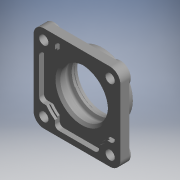
# Autodesk Inventor part: FY 506 M-housing
Saved by Autodesk Inventor 2017.3 (Build 213256000, 256)
## iProperties
Part Number: FY 506 M-housing
Material: Generic
Catalog Web Link: www.cadenas.de
Description: ayf_001hc_hh_hy-housing-Square flanged housings for Y-bearings
Vendor: SKF
Document SubType Name: Modeling
Designer: partserver
Manufacturer: SKF
Mass: 106.222 g
Surface Area: 357.74 cm^2
Volume: 106.222 cm^3
Density: 1 g/cm^3
Appearance: PSOLRGB-175-175-175
Category: PARTsolutions
Company: SKF
Title: FY 506 M-housing
Author: Cadenas PARTsolutions
Comments: Square flanged housings for Y-bearings
PSOL_IDENT_0: {$CADENAS_DATA\23d-libs\skf\bearings_units_and_housings\bearing_units\ball_bearing_units\y-units\y-b
PSOL_IDENT_1: earing_square_flanged_units_parts\ayf_001hc_hh_hy_housing.prj},196 {VTYP=3D},{NB=FY 506 M-housing},{
PSOL_IDENT_2: LINA=FY 506 M-housing},{NN=ayf_001hc_hh_hy-housing},{DATE=20.08.2020 13:45:19},{GEOMDATE=29.07.2020
PSOL_IDENT_3: 16:36:58},{VERSION=},{LINEID=8870},{WBVAR=COVER},{WBNUMERIC=}  {NB=FY 506 M-housing},{LINA=FY 506 M-
PSOL_IDENT_4: housing},{KT=DUMMY},{DESIGNATION=FY 506 M},{SS1=26.700},{T=46.700},{COVER=},{GN=1/4-28 SAE-LT},{D=62
PSOL_IDENT_5: .000},{DA=93.700},{DB1=76.000},{DB2=84.000},{DB=0.000},{A=32.500},{A1=13.000},{A2=20.000},{A3=3.200}
PSOL_IDENT_6: ,{A5=20.000},{J=82.500},{L=108.000},{N=11.500},{RG=1/4-28 UNF},{R1=21.000},{DN=6.500},{SWN=7.000},{J
PSOL_IDENT_7: 6=96.000},{J7=24.500},{N4=4.000},{EC=ECY 206},{AEC=25.000},{DEC=59.400},{D1EC=65.000},{D2EC=66.500},
PSOL_IDENT_8: {E=18},{DESIGN=fy},{BRG=0.000},{ECPN=},{H4=MIN},{R2=MIN},{R3=MIN},{R4=MIN},{L1=MIN},{H5=MIN},{R5=MIN
PSOL_IDENT_9: },{H6=MIN},{L2=MIN},{H7=MIN},{H8=MIN},{H9=MIN},{L3=MIN},{L4=MIN},{H10=MIN},{H11=MIN},{H12=MIN},{H13=
PSOL_IDENT_10: MIN},{H14=MIN},{R6=MIN},{L5=MIN},{H15=MIN},{H16=MIN},{SC=MIN}
NB: FY 506 M-housing
NN: ayf_001hc_hh_hy-housing
NT: Square flanged housings for Y-bearings
NBSYN: $DESIGNATION.$ECPN.-housing
LINA: FY 506 M-housing
CATALOG: SKF
DESIGNATION: FY 506 M
SS1: 26.7
T: 46.7
COVER: No End Cover
GN: 1/4-28 SAE-LT
D: 62
DA: 93.7
DB1: 76
DB2: 84
DB: 0
A: 32.5
A1: 13
A2: 20
A3: 3.2
A5: 20
J: 82.5
L: 108
N: 11.5
RG: 1/4-28 UNF
R1: 21
DN: 6.5
SWN: 7
J6: 96
J7: 24.5
N4: 4
EC: ECY 206
AEC: 25
DEC: 59.4
D1EC: 65
D2EC: 66.5
DESIGN: fy
H4: 0
R2: 0
R3: 0
R4: 0
L1: 0
H5: 0
R5: 0
H6: 0
L2: 0
H7: 0
H8: 0
H9: 0
L3: 0
L4: 0
H10: 0
H11: 0
H12: 0
H13: 0
H14: 0
R6: 0
L5: 0
H15: 0
H16: 0
SC: 0
SUPPLIER: SKF
ARTICLENO: FY 506 M-housing
BOMINFO: FY 506 M-housing
CREATOR: CADENAS GmbH
Autodesk Inventor part; units mm, degrees
sketch "Sketch_1" plane through (0, 0, 0) normal (0, 0, 1) x (1, 0, 0)
  line L0 (0, 0) -> (0, 32.5)
  line L1 (29.6648, 9) -> (32.6648, 6)
  line L2 (32.6648, 6) -> (44.991, 6)
  line L3 (44.991, 6) -> (44.991, 3.2)
  line L4 (44.991, 3.2) -> (46.85, 3.2)
  line L5 (46.85, 3.2) -> (46.85, 0)
  line L6 (46.85, 0) -> (76.3675, 0)
  line L7 (76.3675, 0) -> (76.3675, 11)
  line L8 (76.3675, 11) -> (45, 11)
  arc A0 (42.0754, 13.3318) -> (45, 11) centre (45, 14) ccw
  line L9 (42.0754, 13.3318) -> (37.9623, 31.3341)
  arc A1 (37.9623, 31.3341) -> (36.5, 32.5) centre (36.5, 31) ccw
  line L10 (36.5, 32.5) -> (31, 32.5)
  line L11 (31, 32.5) -> (31, 30.3352)
  line L12 (31, 30.3352) -> (29.6648, 29)
  arc A2 (29.6648, 11) -> (29.6648, 29) centre (0, 20) ccw
  line L13 (29.6648, 11) -> (29.6648, 9)
  constraints: 28 end point, 6 point on circle, 3 centre point
revolve "Revolution1" add sketch "Sketch_1" angle 360 about axis through (0, 0, 0) along (0, -1, 0)
sketch "Sketch_2" plane through (0, 11, 0) normal (0, 1, 0) x (1, 0, 0)
  arc A0 (-50.2656, -32.2344) -> (-32.2344, -50.2656) centre (-41.25, -41.25) ccw
  line L0 (-32.2344, -50.2656) -> (-19.2814, -37.3126)
  arc A1 (-19.2814, -37.3126) -> (19.2814, -37.3126) centre (0, 0) ccw
  line L1 (19.2814, -37.3126) -> (32.2344, -50.2656)
  arc A2 (32.2344, -50.2656) -> (50.2656, -32.2344) centre (41.25, -41.25) ccw
  line L2 (50.2656, -32.2344) -> (37.3126, -19.2814)
  arc A3 (37.3126, -19.2814) -> (37.3126, 19.2814) centre (0, 0) ccw
  line L3 (37.3126, 19.2814) -> (50.2656, 32.2344)
  arc A4 (50.2656, 32.2344) -> (32.2344, 50.2656) centre (41.25, 41.25) ccw
  line L4 (32.2344, 50.2656) -> (19.2814, 37.3126)
  arc A5 (19.2814, 37.3126) -> (-19.2814, 37.3126) centre (0, 0) ccw
  line L5 (-19.2814, 37.3126) -> (-32.2344, 50.2656)
  arc A6 (-32.2344, 50.2656) -> (-50.2656, 32.2344) centre (-41.25, 41.25) ccw
  line L6 (-50.2656, 32.2344) -> (-37.3126, 19.2814)
  arc A7 (-37.3126, 19.2814) -> (-37.3126, -19.2814) centre (0, 0) ccw
  line L7 (-37.3126, -19.2814) -> (-50.2656, -32.2344)
  circle A8 centre (0, 0) radius 41.5
  constraints: 16 end point, 16 point on circle, 9 centre point
extrude "Extrusion1" add sketch "Sketch_2" along normal blind 2
sketch "Sketch_3" plane through (0, 0, 0) normal (0, 1, 0) x (-1, 0, 0)
  line L0 (108, -108) -> (108, 108)
  line L1 (108, 108) -> (-108, 108)
  line L2 (-108, 108) -> (-108, -108)
  line L3 (-108, -108) -> (108, -108)
  arc A0 (54, 41.25) -> (41.25, 54) centre (41.25, 41.25) ccw
  line L4 (41.25, 54) -> (-41.25, 54)
  arc A1 (-41.25, 54) -> (-54, 41.25) centre (-41.25, 41.25) ccw
  line L5 (-54, 41.25) -> (-54, -41.25)
  arc A2 (-54, -41.25) -> (-41.25, -54) centre (-41.25, -41.25) ccw
  line L6 (-41.25, -54) -> (41.25, -54)
  arc A3 (41.25, -54) -> (54, -41.25) centre (41.25, -41.25) ccw
  line L7 (54, -41.25) -> (54, 41.25)
  constraints: 16 end point, 8 point on circle, 4 centre point
extrude "Extrusion2" cut sketch "Sketch_3" along normal blind 32.5
sketch "Sketch4" plane through (-41.25, 0, -54) normal (0, -1, 0) x (1, 0, 0)
  point P0 (0, 95.25)
hole "Hole1" at (-41.25, 0, 41.25) direction (0, 1, 0) diameter 11.5 depth 13
pattern_linear "Rectangular Pattern1" count 2 spacing 82.5 along (1, 0, 0) count 2 spacing 82.5 along (0, 0, -1) of "Hole1"
sketch "Sketch_8" plane through (0, 0, 0) normal (1, 0, 0) x (0, 1, 0)
  line L0 (21, -40.3234) -> (14.0953, -10.1021)
  line L1 (14.0953, -10.1021) -> (17.1905, -9.3949)
  line L2 (17.1905, -9.3949) -> (24.0952, -39.6162)
  line L3 (24.0952, -39.6162) -> (21, -40.3234)
  line L4 (21, -40.3234) -> (14.0953, -10.1021)
  constraints: 10 end point
revolve "Revolution2" cut sketch "Sketch_8" angle 360 about axis through (0, 21, -40.3234) along (0, 0.2227338, -0.9748793)
sketch "Sketch_6" plane through (0, 11, 0) normal (0, 1, 0) x (1, 0, 0)
  line L0 (-50, -24.5) -> (50, -24.5)
  arc A0 (-50, -24.5) -> (-46, -24.5) centre (-48, -24.5) ccw
  line L1 (-50, -24.5) -> (-46, -24.5)
  constraints: 4 end point, 2 point on circle, 1 centre point
revolve "Revolution3" cut sketch "Sketch_6" angle 360 about axis through (-50, 11, 24.5) along (-1, 0, 0)
sketch "Sketch_17" plane through (0, 0, 0) normal (0, 0, 1) x (1, 0, 0)
  line L0 (0, 0) -> (0, 32.5)
  line L1 (27, 26.8511) -> (27, 14.1493)
  line L2 (27, 14.1493) -> (33.5, 17.9021)
  arc A0 (33.5, 17.9021) -> (33.5, 23.0983) centre (32, 20.5002) ccw
  line L3 (33.5, 23.0983) -> (27, 26.8511)
  constraints: 8 end point, 2 point on circle, 1 centre point
revolve "Revolution4" cut sketch "Sketch_17" angle 360 about axis through (0, 0, 0) along (0, -1, 0)
sketch "Sketch_7" plane through (0, 20, 0) normal (0, 1, 0) x (1, 0, 0)
  arc A0 (-27.4003, 14.499) -> (-27.4003, -14.499) centre (0, 0) ccw
  line L0 (-27.4003, -14.499) -> (27.4003, -14.499)
  arc A1 (27.4003, -14.499) -> (27.4003, 14.499) centre (0, 0) ccw
  line L1 (27.4003, 14.499) -> (-27.4003, 14.499)
  constraints: 4 end point, 4 point on circle, 2 centre point
extrude "Extrusion3" cut sketch "Sketch_7" along normal blind 13.975
sketch "Sketch_11" plane through (0, 0, 0) normal (0, 1, 0) x (-1, 0, 0)
  arc A0 (47, 22.45) -> (42, 27.45) centre (42, 22.45) ccw
  line L0 (42, 27.45) -> (27.45, 27.45)
  line L1 (27.45, 27.45) -> (27.45, 42)
  arc A1 (27.45, 42) -> (22.45, 47) centre (22.45, 42) ccw
  line L2 (22.45, 47) -> (-22.45, 47)
  arc A2 (-22.45, 47) -> (-27.45, 42) centre (-22.45, 42) ccw
  line L3 (-27.45, 42) -> (-27.45, 27.45)
  line L4 (-27.45, 27.45) -> (-42, 27.45)
  arc A3 (-42, 27.45) -> (-47, 22.45) centre (-42, 22.45) ccw
  line L5 (-47, 22.45) -> (-47, -22.45)
  arc A4 (-47, -22.45) -> (-42, -27.45) centre (-42, -22.45) ccw
  line L6 (-42, -27.45) -> (-27.45, -27.45)
  line L7 (-27.45, -27.45) -> (-27.45, -42)
  arc A5 (-27.45, -42) -> (-22.45, -47) centre (-22.45, -42) ccw
  line L8 (-22.45, -47) -> (22.45, -47)
  arc A6 (22.45, -47) -> (27.45, -42) centre (22.45, -42) ccw
  line L9 (27.45, -42) -> (27.45, -27.45)
  line L10 (27.45, -27.45) -> (42, -27.45)
  arc A7 (42, -27.45) -> (47, -22.45) centre (42, -22.45) ccw
  line L11 (47, -22.45) -> (47, 22.45)
  constraints: 24 end point, 16 point on circle, 8 centre point
extrude "Extrusion4" cut sketch "Sketch_11" along normal blind 6
sketch "Sketch_12" plane through (0, 11, 0) normal (0, 1, 0) x (1, 0, 0)
  arc A0 (-52.5, 4.7066) -> (-52.2623, 4.4689) centre (-52.2623, 4.7066) ccw
  line L0 (-52.2623, 4.4689) -> (-50.6968, 4.4689)
  arc A1 (-50.6968, 4.4689) -> (-50.5287, 4.5385) centre (-50.6968, 4.7066) ccw
  line L1 (-50.5287, 4.5385) -> (-50.4595, 4.6077)
  arc A2 (-50.2207, 4.7066) -> (-50.4595, 4.6077) centre (-50.2207, 4.3689) ccw
  line L2 (-50.2207, 4.7066) -> (-49.0328, 4.7066)
  arc A3 (-48.8648, 4.637) -> (-49.0328, 4.7066) centre (-49.0328, 4.4689) ccw
  line L3 (-48.8648, 4.637) -> (-48.7663, 4.5385)
  arc A4 (-48.7663, 4.5385) -> (-48.5982, 4.4689) centre (-48.5982, 4.7066) ccw
  line L4 (-48.5982, 4.4689) -> (-47.2704, 4.4689)
  line L5 (-47.2704, 4.4689) -> (-47.2704, 3.732)
  line L6 (-47.2704, 3.732) -> (-48.6967, 3.732)
  arc A5 (-48.6967, 3.732) -> (-48.9344, 3.4943) centre (-48.6967, 3.4943) ccw
  line L7 (-48.9344, 3.4943) -> (-48.9344, 1.9183)
  arc A6 (-48.9916, 1.7636) -> (-48.9344, 1.9183) centre (-49.1721, 1.9183) ccw
  line L8 (-48.9916, 1.7636) -> (-50.3606, 0.1664)
  line L9 (-50.3606, 0.1664) -> (-51.0041, 0.8099)
  arc A7 (-51.0738, 0.978) -> (-51.0041, 0.8099) centre (-50.836, 0.978) ccw
  line L10 (-51.0738, 0.978) -> (-51.0738, 2.7812)
  arc A8 (-51.0738, 2.7812) -> (-51.3115, 3.0189) centre (-51.3115, 2.7812) ccw
  line L11 (-51.3115, 3.0189) -> (-52.2623, 3.0189)
  arc A9 (-52.2623, 3.0189) -> (-52.5, 2.7812) centre (-52.2623, 2.7812) ccw
  line L12 (-52.5, 2.7812) -> (-52.5, 0.7486)
  arc A10 (-52.5, 0.7486) -> (-52.4202, 0.5709) centre (-52.2623, 0.7486) ccw
  line L13 (-52.4202, 0.5709) -> (-50.3606, -1.2599)
  line L14 (-50.3606, -1.2599) -> (-52.2623, -1.2599)
  arc A11 (-52.2623, -1.2599) -> (-52.5, -1.4976) centre (-52.2623, -1.4976) ccw
  line L15 (-52.5, -1.4976) -> (-52.5, -3.3992)
  arc A12 (-52.5, -3.3992) -> (-52.2623, -3.6369) centre (-52.2623, -3.3992) ccw
  line L16 (-52.2623, -3.6369) -> (-50.6968, -3.6369)
  arc A13 (-50.6968, -3.6369) -> (-50.5287, -3.5673) centre (-50.6968, -3.3992) ccw
  line L17 (-50.5287, -3.5673) -> (-50.4302, -3.4689)
  arc A14 (-50.2622, -3.3992) -> (-50.4302, -3.4689) centre (-50.2622, -3.6369) ccw
  line L18 (-50.2622, -3.3992) -> (-49.2705, -3.3992)
  arc A15 (-49.1025, -3.4689) -> (-49.2705, -3.3992) centre (-49.2705, -3.6369) ccw
  line L19 (-49.1025, -3.4689) -> (-49.004, -3.5673)
  arc A16 (-49.004, -3.5673) -> (-48.8359, -3.6369) centre (-48.8359, -3.3992) ccw
  line L20 (-48.8359, -3.6369) -> (-47.2704, -3.6369)
  line L21 (-47.2704, -3.6369) -> (-47.2704, -4.1124)
  line L22 (-47.2704, -4.1124) -> (-50.1229, -4.1124)
  arc A17 (-50.1229, -4.1124) -> (-50.3606, -4.3501) centre (-50.1229, -4.3501) ccw
  line L23 (-50.3606, -4.3501) -> (-50.3606, -8.1534)
  arc A18 (-50.5983, -8.3911) -> (-50.3606, -8.1534) centre (-50.5983, -8.1534) ccw
  line L24 (-50.5983, -8.3911) -> (-51.5492, -8.3911)
  arc A19 (-51.7869, -8.1534) -> (-51.5492, -8.3911) centre (-51.5492, -8.1534) ccw
  line L25 (-51.7869, -8.1534) -> (-51.7869, -7.2026)
  arc A20 (-51.5492, -6.9649) -> (-51.7869, -7.2026) centre (-51.5492, -7.2026) ccw
  line L26 (-51.5492, -6.9649) -> (-51.3115, -6.9649)
  arc A21 (-51.3115, -6.9649) -> (-51.0738, -6.7271) centre (-51.3115, -6.7271) ccw
  line L27 (-51.0738, -6.7271) -> (-51.0738, -5.0632)
  arc A22 (-51.0738, -5.0632) -> (-51.3115, -4.8255) centre (-51.3115, -5.0632) ccw
  line L28 (-51.3115, -4.8255) -> (-52.1923, -4.8255)
  arc A23 (-52.1923, -4.8255) -> (-52.5, -5.1332) centre (-52.1923, -5.1332) ccw
  line L29 (-52.5, -5.1332) -> (-52.5, -10.2428)
  arc A24 (-52.5, -10.2428) -> (-52.2123, -10.5305) centre (-52.2123, -10.2428) ccw
  line L30 (-52.2123, -10.5305) -> (-49.8852, -10.5305)
  arc A25 (-49.8852, -10.5305) -> (-49.6475, -10.2928) centre (-49.8852, -10.2928) ccw
  line L31 (-49.6475, -10.2928) -> (-49.6475, -6.4894)
  arc A26 (-49.4098, -6.2517) -> (-49.6475, -6.4894) centre (-49.4098, -6.4894) ccw
  line L32 (-49.4098, -6.2517) -> (-47.7458, -6.2517)
  arc A27 (-47.5081, -6.4894) -> (-47.7458, -6.2517) centre (-47.7458, -6.4894) ccw
  line L33 (-47.5081, -6.4894) -> (-47.5081, -8.8665)
  arc A28 (-47.7458, -9.1042) -> (-47.5081, -8.8665) centre (-47.7458, -8.8665) ccw
  line L34 (-47.7458, -9.1042) -> (-48.6967, -9.1042)
  arc A29 (-48.6967, -9.1042) -> (-48.9344, -9.3419) centre (-48.6967, -9.3419) ccw
  line L35 (-48.9344, -9.3419) -> (-48.9344, -11.0059)
  arc A30 (-48.9344, -11.0059) -> (-48.6967, -11.2436) centre (-48.6967, -11.0059) ccw
  line L36 (-48.6967, -11.2436) -> (-47.0327, -11.2436)
  arc A31 (-47.0327, -11.2436) -> (-46.795, -11.0059) centre (-47.0327, -11.0059) ccw
  line L37 (-46.795, -11.0059) -> (-46.795, -4.3501)
  arc A32 (-46.795, -4.3501) -> (-47.0327, -4.1124) centre (-47.0327, -4.3501) ccw
  line L38 (-47.0327, -4.1124) -> (-47.0327, -3.6369)
  arc A33 (-47.0327, -3.6369) -> (-46.795, -3.3992) centre (-47.0327, -3.3992) ccw
  line L39 (-46.795, -3.3992) -> (-46.795, -1.4976)
  arc A34 (-46.795, -1.4976) -> (-47.0327, -1.2599) centre (-47.0327, -1.4976) ccw
  line L40 (-47.0327, -1.2599) -> (-48.9344, -1.2599)
  line L41 (-48.9344, -1.2599) -> (-46.8646, 0.8099)
  arc A35 (-46.8646, 0.8099) -> (-46.795, 0.978) centre (-47.0327, 0.978) ccw
  line L42 (-46.795, 0.978) -> (-46.795, 3.4943)
  arc A36 (-46.795, 3.4943) -> (-47.0327, 3.732) centre (-47.0327, 3.4943) ccw
  line L43 (-47.0327, 3.732) -> (-47.0327, 4.4689)
  arc A37 (-47.0327, 4.4689) -> (-46.795, 4.7066) centre (-47.0327, 4.7066) ccw
  line L44 (-46.795, 4.7066) -> (-46.795, 6.6083)
  arc A38 (-46.795, 6.6083) -> (-47.0327, 6.846) centre (-47.0327, 6.6083) ccw
  line L45 (-47.0327, 6.846) -> (-48.6967, 6.846)
  arc A39 (-48.6967, 6.846) -> (-48.9344, 6.6083) centre (-48.6967, 6.6083) ccw
  arc A40 (-49.1721, 6.3706) -> (-48.9344, 6.6083) centre (-49.1721, 6.6083) ccw
  line L46 (-49.1721, 6.3706) -> (-49.4098, 6.3706)
  arc A41 (-49.6475, 6.6083) -> (-49.4098, 6.3706) centre (-49.4098, 6.6083) ccw
  line L47 (-49.6475, 6.6083) -> (-49.6475, 7.4607)
  arc A42 (-49.5779, 7.6287) -> (-49.6475, 7.4607) centre (-49.4098, 7.4607) ccw
  line L48 (-49.5779, 7.6287) -> (-49.4794, 7.7272)
  arc A43 (-49.4794, 7.7272) -> (-49.4098, 7.8953) centre (-49.6475, 7.8953) ccw
  line L49 (-49.4098, 7.8953) -> (-49.4098, 9.4608)
  arc A44 (-49.4098, 9.4608) -> (-49.6475, 9.6985) centre (-49.6475, 9.4608) ccw
  line L50 (-49.6475, 9.6985) -> (-50.3606, 9.6985)
  arc A45 (-50.3606, 9.6985) -> (-50.5983, 9.4608) centre (-50.3606, 9.4608) ccw
  line L51 (-50.5983, 9.4608) -> (-50.5983, 7.8953)
  arc A46 (-50.5983, 7.8953) -> (-50.5287, 7.7272) centre (-50.3606, 7.8953) ccw
  line L52 (-50.5287, 7.7272) -> (-50.4302, 7.6287)
  arc A47 (-50.3606, 7.4607) -> (-50.4302, 7.6287) centre (-50.5983, 7.4607) ccw
  line L53 (-50.3606, 7.4607) -> (-50.3606, 6.6083)
  arc A48 (-50.5983, 6.3706) -> (-50.3606, 6.6083) centre (-50.5983, 6.6083) ccw
  line L54 (-50.5983, 6.3706) -> (-51.4492, 6.3706)
  arc A49 (-51.7869, 6.7083) -> (-51.4492, 6.3706) centre (-51.4492, 6.7083) ccw
  line L55 (-51.7869, 6.7083) -> (-51.7869, 8.7477)
  arc A50 (-51.5492, 8.9854) -> (-51.7869, 8.7477) centre (-51.5492, 8.7477) ccw
  line L56 (-51.5492, 8.9854) -> (-51.3115, 8.9854)
  arc A51 (-51.3115, 8.9854) -> (-51.0738, 9.2231) centre (-51.3115, 9.2231) ccw
  line L57 (-51.0738, 9.2231) -> (-51.0738, 11.6002)
  arc A52 (-51.0738, 11.6002) -> (-51.3115, 11.8379) centre (-51.3115, 11.6002) ccw
  line L58 (-51.3115, 11.8379) -> (-52.2623, 11.8379)
  arc A53 (-52.2623, 11.8379) -> (-52.5, 11.6002) centre (-52.2623, 11.6002) ccw
  line L59 (-52.5, 11.6002) -> (-52.5, 4.7066)
  constraints: 120 end point, 108 point on circle, 54 centre point
extrude "Extrusion5" add sketch "Sketch_12" along normal blind 0.7
sketch "Sketch_13" plane through (0, 0, 0) normal (0, 0, 1) x (1, 0, 0)
  line L0 (0, 27.5) -> (0, 52.5)
  line L1 (0, 32.5) -> (32.054, 32.5)
  line L2 (32.054, 32.5) -> (32.5, 29.5)
  arc A0 (32.5, 27.5) -> (32.5, 29.5) centre (32.2083, 28.5) ccw
  line L3 (32.5, 27.5) -> (0, 27.5)
  line L4 (0, 27.5) -> (0, 32.5)
  constraints: 10 end point, 2 point on circle, 1 centre point
revolve "Revolution5" cut sketch "Sketch_13" angle 360 about axis through (0, 27.5, 0) along (0, -1, 0)
ref_plane "brg_XY" through (0, 20, 0) normal (0, 1, 0) x (1, 0, 0)
ref_plane "brg_YZ" through (0, 20, 0) normal (1, 0, 0) x (0, 0, -1)
ref_plane "brg_ZX" through (0, 20, 0) normal (0, 0, -1) x (0, 1, 0)
ref_plane "gn_XY" through (0, 21, -40.3234) normal (1, 0, 0) x (0, 0.9848078, 0.1736482)
ref_plane "gn_YZ" through (0, 21, -40.3234) normal (0, 0.9848078, 0.1736482) x (0, -0.1736482, 0.9848078)
ref_plane "gn_ZX" through (0, 21, -40.3234) normal (0, -0.1736482, 0.9848078) x (1, 0, 0)
ref_plane "housing_XY" through (0, 0, 0) normal (0, 1, 0) x (1, 0, 0)
ref_plane "housing_YZ" through (0, 0, 0) normal (1, 0, 0) x (0, 0, -1)
ref_plane "housing_ZX" through (0, 0, 0) normal (0, 0, -1) x (0, 1, 0)
ref_plane "tocover_XY" through (0, 52.5, 0) normal (0, 1, 0) x (1, 0, 0)
ref_plane "tocover_YZ" through (0, 52.5, 0) normal (1, 0, 0) x (0, 0, -1)
ref_plane "tocover_ZX" through (0, 52.5, 0) normal (0, 0, -1) x (0, 1, 0)
body "Solid1"
